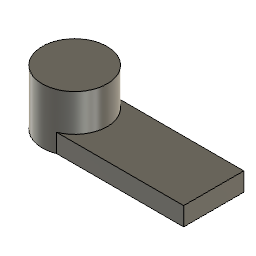
CAP-SCREW (Autodesk Fusion 360 design; units mm, degrees)
part number: 2026-05-20-21-13-29-780
Autodesk Fusion 360 part; units mm, degrees
sketch "Sketch1" plane through (0, 0, 0) normal (0, 0, 1) x (1, 0, 0)
  circle A0 centre (0, 0) radius 3.5
  line L0 (1.299, 3.25) -> (15, 3.25)
  line L1 (15, 3.25) -> (15, -3.25)
  line L2 (15, -3.25) -> (1.299, -3.25)
  line L3 (0, 0) -> (-14.556, 0) construction
  dimension "d1" = 7
  dimension "d2" = 13.701
  dimension "d3" = 6.5
  constraint coincident A0.centre L3.start
  constraint horizontal L0
  constraint vertical L1
  constraint horizontal L2
  constraint coincident A0 L0.start
  constraint horizontal L3
  constraint symmetric L0 L2 L3
  measures "d1" diameter of A0
  measures "d2" distance of L0.start L0.end
  measures "d3" distance of L0.end L1.end
extrude "Extrude1" add sketch "Sketch1" along normal blind 6 contours A0
extrude "Extrude2" add sketch "Sketch1" along normal blind 2 contours A0 L0 L1 L2
